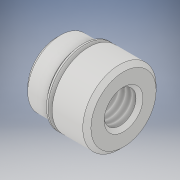
# Autodesk Inventor part: 0070000_rear_head
Saved by Autodesk Inventor 2018 (Build 220112000, 112)
## iProperties
Created: 2019-01-16
Part Number: 0070000_rear_head
Material: Generic
Catalog Web Link: www.cadenas.de
Description: Rear Head-Original Line - Standard Air Cylinders
Vendor: BIMBA
Document SubType Name: Modeling
Designer: s-4008082
Manufacturer: BIMBA
Mass: 0.374422 g
Surface Area: 4.71585 cm^2
Volume: 0.374422 cm^3
Density: 1 g/cm^3
Appearance: PSOLRGB-211-211-211
Category: PARTsolutions
Company: BIMBA
Title: 0070000_rear_head
Author: Cadenas PARTsolutions
Comments: Original Line - Standard Air Cylinders
PSOL_IDENT_0: {$CADENAS_DATA\23d-libs\bimba\bimba\bimba_imperial\bimba_full_line\original_line_cylinders\standard_
PSOL_IDENT_1: air_cylinders\rear_head.prj},239 {VTYP=3D},{NB=0070000_rear_head},{LINA=0070000_rear_head},{NN=Rear
PSOL_IDENT_2: Head},{DATE=21.03.2018 14:31:21},{GEOMDATE=30.06.2014 06:34:00},{VERSION=},{LINEID=10},{WBVAR=MNT,AC
PSOL_IDENT_3: TING,DER,Q,T1,T2,T3,T4,TRIM,Y,K,MB,CUSH,FBON},{WBNUMERIC=TRIM,MB,CUSH}  {NB=0070000_rear_head},{LINA=
PSOL_IDENT_4: 0070000_rear_head},{KT=DUMMY},{PN=0070000},{BORE=0.31250},{BOREPN=007},{MNT=},{MNTALG='' , 'Front No
PSOL_IDENT_5: se' , 'P' , 'Rear Pivot'},{ACTING=},{ACTINGALG= '' , 'Single Acting' },{DER=},{DERALG= '' , 'Standar
PSOL_IDENT_6: d' },{Q=},{T1=},{T2=},{T3=},{T4=},{TRIM=0},{Y=},{K=},{KALG= '', 'without K', 'K', 'with K' },{MB=0},
PSOL_IDENT_7: {A1=0.3280},{A1N=0.3280},{A1P=0.8750},{A1B=0.0000},{A1S=0.0000},{A2=0.1585},{A2N=0.1585},{A3=0.0220}
PSOL_IDENT_8: ,{D1=0.3590},{D1N=0.3590},{D1P=0.4380},{D1B=0.0000},{D2=0.3215},{C1=0.0200},{C2=0.0200},{NDM=0.1900}
PSOL_IDENT_9: ,{TAB=UNF},{NDMDP=0.2000},{D3=0.0000},{A4=0.0000},{A5=0.0000},{D4=0.0000},{A6=0.0000},{A7=0.3750},{A
PSOL_IDENT_10: 8=0.0520},{D5=0.3590},{D6=0.1562},{A9=0.4850},{NDM2=0.3750},{TAB2=UNF},{C11=0.0200},{C22=0.0100},{C3
PSOL_IDENT_11: 3=0.0100},{C44=0.0100},{A10=0.2500},{A11=0.3975},{NDM3=0.1900},{NDM3N=0.1900},{NDM3B=0.0000},{TAB3=U
PSOL_IDENT_12: NF},{TAB3N=UNF},{TAB3B=-},{A12=0.375},{A12N=0.3750},{A12B=0.0000},{A13=0.7190},{D7=0.1270},{D8=0.000
PSOL_IDENT_13: 0},{A14=0.0000},{A15=0.0000},{D9=0.0000},{R1=0.0000},{X1=0.0000},{X2=0.0000},{CX=0.0000},{CC=0.0000}
PSOL_IDENT_14: ,{CON=0},{S1=0.0000},{DB=0.0000},{X1B=0.0000},{X2B=0.0000},{A8B=0.0000},{A9B=0.0000},{MODEL=1},{NDM4=
PSOL_IDENT_15: 0.0000},{TAB4=-},{NDM4DP=0.0000},{BC=0.0000},{B1=0.0000},{B2=0.0000},{B3=0.0000},{ON=0},{ON2=1},{G1=
PSOL_IDENT_16: 0.0000},{G2=0.0000},{G3=0.0000},{G4=0.0000},{GD=0.0000},{G5=0.0000},{G6=0.0000},{RON=0},{H1=0.0000},
PSOL_IDENT_17: {H2=0.0000},{H3=0.0000},{H4=0.0000},{H5=0.0000},{H6=0.0000},{F=0.0000},{PNUT=0.0000},{CUSH=0},{CC11=
PSOL_IDENT_18: 0.000},{CC111=0.0000},{CC22=0.0000},{CC33=0.0000},{CC44=0.0000},{CC55=0.0000},{CD1=0.0000},{CD2=0.00
PSOL_IDENT_19: 00},{CD3=0.0000},{CNDM3=0.0000},{CTAB3=0.0000},{OLEN=0.3280},{OD=0.1895},{STDIS=0.0000},{STDIS1=0.00
PSOL_IDENT_20: 00},{BUSHCON=D-25359},{BUSHL=0.2500},{FBON=0},{LCD=0.0000}
NN: Rear Head
NT: Original Line - Standard Air Cylinders
NB: 0070000_rear_head
NBSYN: $PN._rear_head
LINA: 0070000_rear_head
PN: 0070000
BORE: 0.3125
BOREPN: 007
MNT: Front Nose
MNTALG: '' , 'Front Nose' , 'P' , 'Rear Pivot'
ACTING: Single Acting
DER: Standard
Q: Without Side Ported Rear Head
T1: without T1
T2: without T2
T3: without T3
T4: without T4
TRIM: 0
Y: without Pivot Bushing
K: without K
MB: 0
A1N: 0.328
A1P: 0.875
A1B: 0
A1S: 0
A2N: 0.1585
A3: 0.022
D1N: 0.359
D1P: 0.438
D1B: 0
D2: 0.3215
C1: 0.02
C2: 0.02
TAB: UNF
NDMDP: 0.2
D3: 0
A4: 0
A5: 0
D4: 0
A6: 0
A7: 0.375
A8: 0.052
D5: 0.359
D6: 0.1562
A9: 0.485
NDM2: 0.375
TAB2: UNF
C11: 0.02
C22: 0.01
C33: 0.01
C44: 0.01
A10: 0.25
A11: 0.3975
NDM3N: 0.19
NDM3B: 0
TAB3N: UNF
TAB3B: -
A12N: 0.375
A12B: 0
A13: 0.719
D7: 0.127
D8: 0
A14: 0
A15: 0
D9: 0
R1: 0
X1: 0
X2: 0
CX: 0
CC: 0
S1: 0
DB: 0
X1B: 0
X2B: 0
A8B: 0
A9B: 0
NDM4: 0
TAB4: -
NDM4DP: 0
BC: 0
B1: 0
B2: 0
B3: 0
G1: 0
G2: 0
G3: 0
G4: 0
GD: 0
G5: 0
G6: 0
H2: 0
H3: 0
F: 0
CUSH: 0
CC111: 0
CC22: 0
CC33: 0
CC44: 0
CC55: 0
CD1: 0
CD2: 0
CD3: 0
CNDM3: 0
CTAB3: 0.0000
OD: 0.1895
STDIS1: 0
BUSHCON: D-25359
BUSHL: 0.25
FBON: 0
LCD: 0
SUPPLIER: BIMBA
ARTICLENO: 0070000_rear_head
BOMINFO: 0070000_rear_head
CREATOR: CADENAS GmbH
Autodesk Inventor part; units mm, degrees
sketch "Sketch_1" plane through (0, 0, 0) normal (0, 0, 1) x (1, 0, 0)
  line L0 (8.3312, 0) -> (0, 0)
  line L1 (0, 0) -> (0, 3.5751)
  line L2 (0, 3.5751) -> (0.508, 4.0831)
  line L3 (0.508, 4.0831) -> (2.9083, 4.0831)
  line L4 (2.9083, 4.0831) -> (3.4671, 3.5242)
  line L5 (3.4671, 3.5242) -> (4.0259, 3.5242)
  line L6 (4.0259, 3.5242) -> (4.0259, 4.5593)
  line L7 (4.0259, 4.5593) -> (7.8232, 4.5593)
  line L8 (7.8232, 4.5593) -> (8.3312, 4.0513)
  line L9 (8.3312, 4.0513) -> (8.3312, 0)
  line L10 (8.3312, 0) -> (0, 0)
  constraints: 22 end point
revolve "Revolution1" add sketch "Sketch_1" angle 360 about axis through (8.3312, 0, 0) along (1, 0, 0)
sketch "Sketch_2" plane through (0, 0, 0) normal (0, 0, 1) x (1, 0, 0)
  line L0 (8.3312, 0) -> (0, 0)
  line L1 (0, 0) -> (0, 2.413)
  line L2 (0, 2.413) -> (0.4293, 1.9837)
  line L3 (0.4293, 1.9837) -> (7.9019, 1.9837)
  line L4 (7.9019, 1.9837) -> (8.3312, 2.413)
  line L5 (8.3312, 2.413) -> (8.3312, 0)
  line L6 (8.3312, 0) -> (0, 0)
  constraints: 14 end point
revolve "Revolution2" cut sketch "Sketch_2" angle 360 about axis through (8.3312, 0, 0) along (1, 0, 0)
thread "Thread1" size "10-32 UNF" class "2B" standard "ANSI Unified Screw Threads" full length
sketch "Sketch_24" plane through (0, 0, 0) normal (0, 0, 1) x (1, 0, 0)
  line L0 (4.0259, 0) -> (3.4671, 0)
  line L1 (3.3065, 4.5593) -> (3.3065, 4.4751)
  line L2 (3.3065, 4.4751) -> (3.9121, 3.8695)
  arc A0 (3.9121, 3.6899) -> (3.9121, 3.8695) centre (3.8223, 3.7797) ccw
  line L3 (3.9121, 3.6899) -> (3.7465, 3.5242)
  line L4 (3.7465, 3.5242) -> (3.4671, 3.5242)
  line L5 (3.4671, 3.5242) -> (3.4671, 3.2702)
  line L6 (3.4671, 3.2702) -> (4.0259, 3.2702)
  line L7 (4.0259, 3.2702) -> (4.0259, 4.0431)
  line L8 (4.0259, 4.0431) -> (3.5097, 4.5593)
  line L9 (3.5097, 4.5593) -> (3.3065, 4.5593)
  constraints: 20 end point, 2 point on circle, 1 centre point
revolve "Revolution3" add sketch "Sketch_24" angle 360 about axis through (4.0259, 0, 0) along (1, 0, 0)
ref_plane "lovra_XY" through (8.3312, 0, 0) normal (1, 0, 0) x (0, 1, 0)
ref_plane "lovra_YZ" through (8.3312, 0, 0) normal (0, 1, 0) x (0, 0, 1)
ref_plane "lovra_ZX" through (8.3312, 0, 0) normal (0, 0, 1) x (1, 0, 0)
ref_plane "lovra1_XY" through (8.3312, 0, 0) normal (1, 0, 0) x (0, 0, -1)
ref_plane "lovra1_YZ" through (8.3312, 0, 0) normal (0, 0, -1) x (0, 1, 0)
ref_plane "lovra1_ZX" through (8.3312, 0, 0) normal (0, 1, 0) x (1, 0, 0)
ref_plane "lovra2_XY" through (8.3312, 0, 0) normal (1, 0, 0) x (0, 0, -1)
ref_plane "lovra2_YZ" through (8.3312, 0, 0) normal (0, 0, -1) x (0, 1, 0)
ref_plane "lovra2_ZX" through (8.3312, 0, 0) normal (0, 1, 0) x (1, 0, 0)
ref_plane "lovra21_XY" through (0, 0, 5.2705) normal (1, 0, 0) x (0, 0, -1)
ref_plane "lovra21_YZ" through (0, 0, 5.2705) normal (0, 0, -1) x (0, 1, 0)
ref_plane "lovra21_ZX" through (0, 0, 5.2705) normal (0, 1, 0) x (1, 0, 0)
ref_plane "lovra22_XY" through (0, 0, -5.2705) normal (1, 0, 0) x (0, 0, -1)
ref_plane "lovra22_YZ" through (0, 0, -5.2705) normal (0, 0, -1) x (0, 1, 0)
ref_plane "lovra22_ZX" through (0, 0, -5.2705) normal (0, 1, 0) x (1, 0, 0)
ref_plane "lovra3_XY" through (8.3312, 0, 0) normal (1, 0, 0) x (0, 0, -1)
ref_plane "lovra3_YZ" through (8.3312, 0, 0) normal (0, 0, -1) x (0, 1, 0)
ref_plane "lovra3_ZX" through (8.3312, 0, 0) normal (0, 1, 0) x (1, 0, 0)
ref_plane "olen_XY" through (8.3312, 0, 0) normal (1, 0, 0) x (0, 0, -1)
ref_plane "olen_YZ" through (8.3312, 0, 0) normal (0, 0, -1) x (0, 1, 0)
ref_plane "olen_ZX" through (8.3312, 0, 0) normal (0, 1, 0) x (1, 0, 0)
ref_plane "to_mounting_bracket_XY" through (13.5509, 0, 0) normal (1, 0, 0) x (0, 0, -1)
ref_plane "to_mounting_bracket_YZ" through (13.5509, 0, 0) normal (0, 0, -1) x (0, 1, 0)
ref_plane "to_mounting_bracket_ZX" through (13.5509, 0, 0) normal (0, 1, 0) x (1, 0, 0)
ref_plane "to_nut_XY" through (0, 0, 0) normal (1, 0, 0) x (0, 0, -1)
ref_plane "to_nut_YZ" through (0, 0, 0) normal (0, 0, -1) x (0, 1, 0)
ref_plane "to_nut_ZX" through (0, 0, 0) normal (0, 1, 0) x (1, 0, 0)
ref_plane "to_pin_XY" through (18.2626, 0, 0) normal (0, 0, 1) x (1, 0, 0)
ref_plane "to_pin_YZ" through (18.2626, 0, 0) normal (1, 0, 0) x (0, 1, 0)
ref_plane "to_pin_ZX" through (18.2626, 0, 0) normal (0, 1, 0) x (0, 0, 1)
ref_plane "to_screw_XY" through (9.525, 0, 0) normal (0, 1, 0) x (1, 0, 0)
ref_plane "to_screw_YZ" through (9.525, 0, 0) normal (1, 0, 0) x (0, 0, -1)
ref_plane "to_screw_ZX" through (9.525, 0, 0) normal (0, 0, -1) x (0, 1, 0)
ref_plane "to_tube_XY" through (3.4671, 0, 0) normal (1, 0, 0) x (0, 0, -1)
ref_plane "to_tube_YZ" through (3.4671, 0, 0) normal (0, 0, -1) x (0, 1, 0)
ref_plane "to_tube_ZX" through (3.4671, 0, 0) normal (0, 1, 0) x (1, 0, 0)
body "Solid1"
